Autodesk Fusion 360 part; units mm, degrees
(part 2 of 4)
sketch "Sketch4" plane through (0, 20, 0) normal (0, 1, 0) x (-1, 0, 0)
  line L0 (95, -45) -> (95, 155)
  line L1 (95, 155) -> (-95, 155)
  line L2 (-95, 155) -> (-95, -45)
  line L3 (-95, -45) -> (95, -45)
  line L4 (-63.1566, 125.0807) -> (-65.6424, 118.6138)
  line L5 (-65.6424, 118.6138) -> (-72.4858, 117.5331)
  line L6 (-72.4858, 117.5331) -> (-76.8434, 122.9193)
  line L7 (-76.8434, 122.9193) -> (-74.3576, 129.3862)
  line L8 (-74.3576, 129.3862) -> (-67.5142, 130.4669)
  line L9 (-67.5142, 130.4669) -> (-63.1566, 125.0807)
  line L10 (-63.1566, 93.0807) -> (-65.6424, 86.6138)
  line L11 (-65.6424, 86.6138) -> (-72.4858, 85.5331)
  line L12 (-72.4858, 85.5331) -> (-76.8434, 90.9193)
  line L13 (-76.8434, 90.9193) -> (-74.3576, 97.3862)
  line L14 (-74.3576, 97.3862) -> (-67.5142, 98.4669)
  line L15 (-67.5142, 98.4669) -> (-63.1566, 93.0807)
  line L16 (-63.1566, 61.0807) -> (-65.6424, 54.6138)
  line L17 (-65.6424, 54.6138) -> (-72.4858, 53.5331)
  line L18 (-72.4858, 53.5331) -> (-76.8434, 58.9193)
  line L19 (-76.8434, 58.9193) -> (-74.3576, 65.3862)
  line L20 (-74.3576, 65.3862) -> (-67.5142, 66.4669)
  line L21 (-67.5142, 66.4669) -> (-63.1566, 61.0807)
  line L22 (-63.1566, 29.0807) -> (-65.6424, 22.6138)
  line L23 (-65.6424, 22.6138) -> (-72.4858, 21.5331)
  line L24 (-72.4858, 21.5331) -> (-76.8434, 26.9193)
  line L25 (-76.8434, 26.9193) -> (-74.3576, 33.3862)
  line L26 (-74.3576, 33.3862) -> (-67.5142, 34.4669)
  line L27 (-67.5142, 34.4669) -> (-63.1566, 29.0807)
  line L28 (-63.1566, -2.9193) -> (-65.6424, -9.3862)
  line L29 (-65.6424, -9.3862) -> (-72.4858, -10.4669)
  line L30 (-72.4858, -10.4669) -> (-76.8434, -5.0807)
  line L31 (-76.8434, -5.0807) -> (-74.3576, 1.3862)
  line L32 (-74.3576, 1.3862) -> (-67.5142, 2.4669)
  line L33 (-67.5142, 2.4669) -> (-63.1566, -2.9193)
  line L34 (-49.8233, 141.0807) -> (-52.3091, 134.6138)
  line L35 (-52.3091, 134.6138) -> (-59.1525, 133.5331)
  line L36 (-59.1525, 133.5331) -> (-63.5101, 138.9193)
  line L37 (-63.5101, 138.9193) -> (-61.0243, 145.3862)
  line L38 (-61.0243, 145.3862) -> (-54.1809, 146.4669)
  line L39 (-54.1809, 146.4669) -> (-49.8233, 141.0807)
  line L40 (-49.8233, 109.0807) -> (-52.3091, 102.6138)
  line L41 (-52.3091, 102.6138) -> (-59.1525, 101.5331)
  line L42 (-59.1525, 101.5331) -> (-63.5101, 106.9193)
  line L43 (-63.5101, 106.9193) -> (-61.0243, 113.3862)
  line L44 (-61.0243, 113.3862) -> (-54.1809, 114.4669)
  line L45 (-54.1809, 114.4669) -> (-49.8233, 109.0807)
  line L46 (-49.8233, 77.0807) -> (-52.3091, 70.6138)
  line L47 (-52.3091, 70.6138) -> (-59.1525, 69.5331)
  line L48 (-59.1525, 69.5331) -> (-63.5101, 74.9193)
  line L49 (-63.5101, 74.9193) -> (-61.0243, 81.3862)
  line L50 (-61.0243, 81.3862) -> (-54.1809, 82.4669)
  line L51 (-54.1809, 82.4669) -> (-49.8233, 77.0807)
  line L52 (-49.8233, 45.0807) -> (-52.3091, 38.6138)
  line L53 (-52.3091, 38.6138) -> (-59.1525, 37.5331)
  line L54 (-59.1525, 37.5331) -> (-63.5101, 42.9193)
  line L55 (-63.5101, 42.9193) -> (-61.0243, 49.3862)
  line L56 (-61.0243, 49.3862) -> (-54.1809, 50.4669)
  line L57 (-54.1809, 50.4669) -> (-49.8233, 45.0807)
  line L58 (-49.8233, 13.0807) -> (-52.3091, 6.6138)
  line L59 (-52.3091, 6.6138) -> (-59.1525, 5.5331)
  line L60 (-59.1525, 5.5331) -> (-63.5101, 10.9193)
  line L61 (-63.5101, 10.9193) -> (-61.0243, 17.3862)
  line L62 (-61.0243, 17.3862) -> (-54.1809, 18.4669)
  line L63 (-54.1809, 18.4669) -> (-49.8233, 13.0807)
  line L64 (-49.8233, -18.9193) -> (-52.3091, -25.3862)
  line L65 (-52.3091, -25.3862) -> (-59.1525, -26.4669)
  line L66 (-59.1525, -26.4669) -> (-63.5101, -21.0807)
  line L67 (-63.5101, -21.0807) -> (-61.0243, -14.6138)
  line L68 (-61.0243, -14.6138) -> (-54.1809, -13.5331)
  line L69 (-54.1809, -13.5331) -> (-49.8233, -18.9193)
  line L70 (-36.4899, 125.0807) -> (-38.9757, 118.6138)
  line L71 (-38.9757, 118.6138) -> (-45.8191, 117.5331)
  line L72 (-45.8191, 117.5331) -> (-50.1767, 122.9193)
  line L73 (-50.1767, 122.9193) -> (-47.6909, 129.3862)
  line L74 (-47.6909, 129.3862) -> (-40.8475, 130.4669)
  line L75 (-40.8475, 130.4669) -> (-36.4899, 125.0807)
  line L76 (-36.4899, 93.0807) -> (-38.9757, 86.6138)
  line L77 (-38.9757, 86.6138) -> (-45.8191, 85.5331)
  line L78 (-45.8191, 85.5331) -> (-50.1767, 90.9193)
  line L79 (-50.1767, 90.9193) -> (-47.6909, 97.3862)
  line L80 (-47.6909, 97.3862) -> (-40.8475, 98.4669)
  line L81 (-40.8475, 98.4669) -> (-36.4899, 93.0807)
  line L82 (-36.4899, 61.0807) -> (-38.9757, 54.6138)
  line L83 (-38.9757, 54.6138) -> (-45.8191, 53.5331)
  line L84 (-45.8191, 53.5331) -> (-50.1767, 58.9193)
  line L85 (-50.1767, 58.9193) -> (-47.6909, 65.3862)
  line L86 (-47.6909, 65.3862) -> (-40.8475, 66.4669)
  line L87 (-40.8475, 66.4669) -> (-36.4899, 61.0807)
  line L88 (-36.4899, 29.0807) -> (-38.9757, 22.6138)
  line L89 (-38.9757, 22.6138) -> (-45.8191, 21.5331)
  line L90 (-45.8191, 21.5331) -> (-50.1767, 26.9193)
  line L91 (-50.1767, 26.9193) -> (-47.6909, 33.3862)
  line L92 (-47.6909, 33.3862) -> (-40.8475, 34.4669)
  line L93 (-40.8475, 34.4669) -> (-36.4899, 29.0807)
  line L94 (-36.4899, -2.9193) -> (-38.9757, -9.3862)
  line L95 (-38.9757, -9.3862) -> (-45.8191, -10.4669)
  line L96 (-45.8191, -10.4669) -> (-50.1767, -5.0807)
  line L97 (-50.1767, -5.0807) -> (-47.6909, 1.3862)
  line L98 (-47.6909, 1.3862) -> (-40.8475, 2.4669)
  line L99 (-40.8475, 2.4669) -> (-36.4899, -2.9193)
  line L100 (-23.1566, 141.0807) -> (-25.6424, 134.6138)
  line L101 (-25.6424, 134.6138) -> (-32.4858, 133.5331)
  line L102 (-32.4858, 133.5331) -> (-36.8434, 138.9193)
  line L103 (-36.8434, 138.9193) -> (-34.3576, 145.3862)
  line L104 (-34.3576, 145.3862) -> (-27.5142, 146.4669)
  line L105 (-27.5142, 146.4669) -> (-23.1566, 141.0807)
  line L106 (-23.1566, 109.0807) -> (-25.6424, 102.6138)
  line L107 (-25.6424, 102.6138) -> (-32.4858, 101.5331)
  line L108 (-32.4858, 101.5331) -> (-36.8434, 106.9193)
  line L109 (-36.8434, 106.9193) -> (-34.3576, 113.3862)
  line L110 (-34.3576, 113.3862) -> (-27.5142, 114.4669)
  line L111 (-27.5142, 114.4669) -> (-23.1566, 109.0807)
  line L112 (-23.1566, 77.0807) -> (-25.6424, 70.6138)
  line L113 (-25.6424, 70.6138) -> (-32.4858, 69.5331)
  line L114 (-32.4858, 69.5331) -> (-36.8434, 74.9193)
  line L115 (-36.8434, 74.9193) -> (-34.3576, 81.3862)
  line L116 (-34.3576, 81.3862) -> (-27.5142, 82.4669)
  line L117 (-27.5142, 82.4669) -> (-23.1566, 77.0807)
  line L118 (-23.1566, 45.0807) -> (-25.6424, 38.6138)
  line L119 (-25.6424, 38.6138) -> (-32.4858, 37.5331)
  line L120 (-32.4858, 37.5331) -> (-36.8434, 42.9193)
  line L121 (-36.8434, 42.9193) -> (-34.3576, 49.3862)
  line L122 (-34.3576, 49.3862) -> (-27.5142, 50.4669)
  line L123 (-27.5142, 50.4669) -> (-23.1566, 45.0807)
  line L124 (-23.1566, 13.0807) -> (-25.6424, 6.6138)
  line L125 (-25.6424, 6.6138) -> (-32.4858, 5.5331)
  line L126 (-32.4858, 5.5331) -> (-36.8434, 10.9193)
  line L127 (-36.8434, 10.9193) -> (-34.3576, 17.3862)
  line L128 (-34.3576, 17.3862) -> (-27.5142, 18.4669)
  line L129 (-27.5142, 18.4669) -> (-23.1566, 13.0807)
  line L130 (-23.1566, -18.9193) -> (-25.6424, -25.3862)
  line L131 (-25.6424, -25.3862) -> (-32.4858, -26.4669)
  line L132 (-32.4858, -26.4669) -> (-36.8434, -21.0807)
  line L133 (-36.8434, -21.0807) -> (-34.3576, -14.6138)
  line L134 (-34.3576, -14.6138) -> (-27.5142, -13.5331)
  line L135 (-27.5142, -13.5331) -> (-23.1566, -18.9193)
  line L136 (-9.8233, 125.0807) -> (-12.3091, 118.6138)
  line L137 (-12.3091, 118.6138) -> (-19.1525, 117.5331)
  line L138 (-19.1525, 117.5331) -> (-23.5101, 122.9193)
  line L139 (-23.5101, 122.9193) -> (-21.0243, 129.3862)
  line L140 (-21.0243, 129.3862) -> (-14.1809, 130.4669)
  line L141 (-14.1809, 130.4669) -> (-9.8233, 125.0807)
  line L142 (-9.8233, 93.0807) -> (-12.3091, 86.6138)
  line L143 (-12.3091, 86.6138) -> (-19.1525, 85.5331)
  line L144 (-19.1525, 85.5331) -> (-23.5101, 90.9193)
  line L145 (-23.5101, 90.9193) -> (-21.0243, 97.3862)
  line L146 (-21.0243, 97.3862) -> (-14.1809, 98.4669)
  line L147 (-14.1809, 98.4669) -> (-9.8233, 93.0807)
  line L148 (-9.8233, 61.0807) -> (-12.3091, 54.6138)
  line L149 (-12.3091, 54.6138) -> (-19.1525, 53.5331)
  line L150 (-19.1525, 53.5331) -> (-23.5101, 58.9193)
  line L151 (-23.5101, 58.9193) -> (-21.0243, 65.3862)
  line L152 (-21.0243, 65.3862) -> (-14.1809, 66.4669)
  line L153 (-14.1809, 66.4669) -> (-9.8233, 61.0807)
  line L154 (-9.8233, 29.0807) -> (-12.3091, 22.6138)
  line L155 (-12.3091, 22.6138) -> (-19.1525, 21.5331)
  line L156 (-19.1525, 21.5331) -> (-23.5101, 26.9193)
  line L157 (-23.5101, 26.9193) -> (-21.0243, 33.3862)
  line L158 (-21.0243, 33.3862) -> (-14.1809, 34.4669)
  line L159 (-14.1809, 34.4669) -> (-9.8233, 29.0807)
  line L160 (-9.8233, -2.9193) -> (-12.3091, -9.3862)
  line L161 (-12.3091, -9.3862) -> (-19.1525, -10.4669)
  line L162 (-19.1525, -10.4669) -> (-23.5101, -5.0807)
  line L163 (-23.5101, -5.0807) -> (-21.0243, 1.3862)
  line L164 (-21.0243, 1.3862) -> (-14.1809, 2.4669)
  line L165 (-14.1809, 2.4669) -> (-9.8233, -2.9193)
  line L166 (-0.8475, 146.4669) -> (3.5101, 141.0807)
  line L167 (3.5101, 141.0807) -> (1.0243, 134.6138)
  line L168 (1.0243, 134.6138) -> (-5.8191, 133.5331)
  line L169 (-5.8191, 133.5331) -> (-10.1767, 138.9193)
  line L170 (-10.1767, 138.9193) -> (-7.6909, 145.3862)
  line L171 (-7.6909, 145.3862) -> (-0.8475, 146.4669)
  line L172 (-0.8475, 114.4669) -> (3.5101, 109.0807)
  line L173 (3.5101, 109.0807) -> (1.0243, 102.6138)
  line L174 (1.0243, 102.6138) -> (-5.8191, 101.5331)
  line L175 (-5.8191, 101.5331) -> (-10.1767, 106.9193)
  line L176 (-10.1767, 106.9193) -> (-7.6909, 113.3862)
  line L177 (-7.6909, 113.3862) -> (-0.8475, 114.4669)
  line L178 (-0.8475, 82.4669) -> (3.5101, 77.0807)
  line L179 (3.5101, 77.0807) -> (1.0243, 70.6138)
  line L180 (1.0243, 70.6138) -> (-5.8191, 69.5331)
  line L181 (-5.8191, 69.5331) -> (-10.1767, 74.9193)
  line L182 (-10.1767, 74.9193) -> (-7.6909, 81.3862)
  line L183 (-7.6909, 81.3862) -> (-0.8475, 82.4669)
  line L184 (-0.8475, 50.4669) -> (3.5101, 45.0807)
  line L185 (3.5101, 45.0807) -> (1.0243, 38.6138)
  line L186 (1.0243, 38.6138) -> (-5.8191, 37.5331)
  line L187 (-5.8191, 37.5331) -> (-10.1767, 42.9193)
  line L188 (-10.1767, 42.9193) -> (-7.6909, 49.3862)
  line L189 (-7.6909, 49.3862) -> (-0.8475, 50.4669)
  line L190 (-0.8475, 18.4669) -> (3.5101, 13.0807)
  line L191 (3.5101, 13.0807) -> (1.0243, 6.6138)
  line L192 (1.0243, 6.6138) -> (-5.8191, 5.5331)
  line L193 (-5.8191, 5.5331) -> (-10.1767, 10.9193)
  line L194 (-10.1767, 10.9193) -> (-7.6909, 17.3862)
  line L195 (-7.6909, 17.3862) -> (-0.8475, 18.4669)
  line L196 (-0.8475, -13.5331) -> (3.5101, -18.9193)
  line L197 (3.5101, -18.9193) -> (1.0243, -25.3862)
  line L198 (1.0243, -25.3862) -> (-5.8191, -26.4669)
  line L199 (-5.8191, -26.4669) -> (-10.1767, -21.0807)
  line L200 (-10.1767, -21.0807) -> (-7.6909, -14.6138)
  line L201 (-7.6909, -14.6138) -> (-0.8475, -13.5331)
  line L202 (12.4858, 130.4669) -> (16.8434, 125.0807)
  line L203 (16.8434, 125.0807) -> (14.3576, 118.6138)
  line L204 (14.3576, 118.6138) -> (7.5142, 117.5331)
  line L205 (7.5142, 117.5331) -> (3.1566, 122.9193)
  line L206 (3.1566, 122.9193) -> (5.6424, 129.3862)
  line L207 (5.6424, 129.3862) -> (12.4858, 130.4669)
  line L208 (12.4858, 98.4669) -> (16.8434, 93.0807)
  line L209 (16.8434, 93.0807) -> (14.3576, 86.6138)
  line L210 (14.3576, 86.6138) -> (7.5142, 85.5331)
  line L211 (7.5142, 85.5331) -> (3.1566, 90.9193)
  line L212 (3.1566, 90.9193) -> (5.6424, 97.3862)
  line L213 (5.6424, 97.3862) -> (12.4858, 98.4669)
  line L214 (12.4858, 66.4669) -> (16.8434, 61.0807)
  line L215 (16.8434, 61.0807) -> (14.3576, 54.6138)
  line L216 (14.3576, 54.6138) -> (7.5142, 53.5331)
  line L217 (7.5142, 53.5331) -> (3.1566, 58.9193)
  line L218 (3.1566, 58.9193) -> (5.6424, 65.3862)
  line L219 (5.6424, 65.3862) -> (12.4858, 66.4669)
  line L220 (12.4858, 34.4669) -> (16.8434, 29.0807)
  line L221 (16.8434, 29.0807) -> (14.3576, 22.6138)
  line L222 (14.3576, 22.6138) -> (7.5142, 21.5331)
  line L223 (7.5142, 21.5331) -> (3.1566, 26.9193)
  line L224 (3.1566, 26.9193) -> (5.6424, 33.3862)
  line L225 (5.6424, 33.3862) -> (12.4858, 34.4669)
  line L226 (12.4858, 2.4669) -> (16.8434, -2.9193)
  line L227 (16.8434, -2.9193) -> (14.3576, -9.3862)
  line L228 (14.3576, -9.3862) -> (7.5142, -10.4669)
  line L229 (7.5142, -10.4669) -> (3.1566, -5.0807)
  line L230 (3.1566, -5.0807) -> (5.6424, 1.3862)
  line L231 (5.6424, 1.3862) -> (12.4858, 2.4669)
  line L232 (25.8191, 146.4669) -> (30.1767, 141.0807)
  line L233 (30.1767, 141.0807) -> (27.6909, 134.6138)
  line L234 (27.6909, 134.6138) -> (20.8475, 133.5331)
  line L235 (20.8475, 133.5331) -> (16.4899, 138.9193)
  line L236 (16.4899, 138.9193) -> (18.9757, 145.3862)
  line L237 (18.9757, 145.3862) -> (25.8191, 146.4669)
  line L238 (25.8191, 114.4669) -> (30.1767, 109.0807)
  line L239 (30.1767, 109.0807) -> (27.6909, 102.6138)
  line L240 (27.6909, 102.6138) -> (20.8475, 101.5331)
  line L241 (20.8475, 101.5331) -> (16.4899, 106.9193)
  line L242 (16.4899, 106.9193) -> (18.9757, 113.3862)
  line L243 (18.9757, 113.3862) -> (25.8191, 114.4669)
  line L244 (25.8191, 82.4669) -> (30.1767, 77.0807)
  line L245 (30.1767, 77.0807) -> (27.6909, 70.6138)
  line L246 (27.6909, 70.6138) -> (20.8475, 69.5331)
  line L247 (20.8475, 69.5331) -> (16.4899, 74.9193)
  line L248 (16.4899, 74.9193) -> (18.9757, 81.3862)
  line L249 (18.9757, 81.3862) -> (25.8191, 82.4669)
  line L250 (25.8191, 50.4669) -> (30.1767, 45.0807)
  line L251 (30.1767, 45.0807) -> (27.6909, 38.6138)
  line L252 (27.6909, 38.6138) -> (20.8475, 37.5331)
  line L253 (20.8475, 37.5331) -> (16.4899, 42.9193)
  line L254 (16.4899, 42.9193) -> (18.9757, 49.3862)
  line L255 (18.9757, 49.3862) -> (25.8191, 50.4669)
  line L256 (25.8191, 18.4669) -> (30.1767, 13.0807)
  line L257 (30.1767, 13.0807) -> (27.6909, 6.6138)
  line L258 (27.6909, 6.6138) -> (20.8475, 5.5331)
  line L259 (20.8475, 5.5331) -> (16.4899, 10.9193)
  line L260 (16.4899, 10.9193) -> (18.9757, 17.3862)
  line L261 (18.9757, 17.3862) -> (25.8191, 18.4669)
  line L262 (25.8191, -13.5331) -> (30.1767, -18.9193)
  line L263 (30.1767, -18.9193) -> (27.6909, -25.3862)
  line L264 (27.6909, -25.3862) -> (20.8475, -26.4669)
  line L265 (20.8475, -26.4669) -> (16.4899, -21.0807)
  line L266 (16.4899, -21.0807) -> (18.9757, -14.6138)
  line L267 (18.9757, -14.6138) -> (25.8191, -13.5331)
  line L268 (39.1525, 130.4669) -> (43.5101, 125.0807)
  line L269 (43.5101, 125.0807) -> (41.0243, 118.6138)
  line L270 (41.0243, 118.6138) -> (34.1809, 117.5331)
  line L271 (34.1809, 117.5331) -> (29.8233, 122.9193)
  line L272 (29.8233, 122.9193) -> (32.3091, 129.3862)
  line L273 (32.3091, 129.3862) -> (39.1525, 130.4669)
  line L274 (39.1525, 98.4669) -> (43.5101, 93.0807)
  line L275 (43.5101, 93.0807) -> (41.0243, 86.6138)
  line L276 (41.0243, 86.6138) -> (34.1809, 85.5331)
  line L277 (34.1809, 85.5331) -> (29.8233, 90.9193)
  line L278 (29.8233, 90.9193) -> (32.3091, 97.3862)
  line L279 (32.3091, 97.3862) -> (39.1525, 98.4669)
  line L280 (39.1525, 66.4669) -> (43.5101, 61.0807)
  line L281 (43.5101, 61.0807) -> (41.0243, 54.6138)
  line L282 (41.0243, 54.6138) -> (34.1809, 53.5331)
  line L283 (34.1809, 53.5331) -> (29.8233, 58.9193)
  line L284 (29.8233, 58.9193) -> (32.3091, 65.3862)
  line L285 (32.3091, 65.3862) -> (39.1525, 66.4669)
  line L286 (39.1525, 34.4669) -> (43.5101, 29.0807)
  line L287 (43.5101, 29.0807) -> (41.0243, 22.6138)
  line L288 (41.0243, 22.6138) -> (34.1809, 21.5331)
  line L289 (34.1809, 21.5331) -> (29.8233, 26.9193)
  line L290 (29.8233, 26.9193) -> (32.3091, 33.3862)
  line L291 (32.3091, 33.3862) -> (39.1525, 34.4669)
  line L292 (39.1525, 2.4669) -> (43.5101, -2.9193)
  line L293 (43.5101, -2.9193) -> (41.0243, -9.3862)
  line L294 (41.0243, -9.3862) -> (34.1809, -10.4669)
  line L295 (34.1809, -10.4669) -> (29.8233, -5.0807)
  line L296 (29.8233, -5.0807) -> (32.3091, 1.3862)
  line L297 (32.3091, 1.3862) -> (39.1525, 2.4669)
  line L298 (52.4858, 146.4669) -> (56.8434, 141.0807)
  line L299 (56.8434, 141.0807) -> (54.3576, 134.6138)
  line L300 (54.3576, 134.6138) -> (47.5142, 133.5331)
  line L301 (47.5142, 133.5331) -> (43.1566, 138.9193)
  line L302 (43.1566, 138.9193) -> (45.6424, 145.3862)
  line L303 (45.6424, 145.3862) -> (52.4858, 146.4669)
  line L304 (52.4858, 114.4669) -> (56.8434, 109.0807)
  line L305 (56.8434, 109.0807) -> (54.3576, 102.6138)
  line L306 (54.3576, 102.6138) -> (47.5142, 101.5331)
  line L307 (47.5142, 101.5331) -> (43.1566, 106.9193)
  line L308 (43.1566, 106.9193) -> (45.6424, 113.3862)
  line L309 (45.6424, 113.3862) -> (52.4858, 114.4669)
  line L310 (52.4858, 82.4669) -> (56.8434, 77.0807)
  line L311 (56.8434, 77.0807) -> (54.3576, 70.6138)
  line L312 (54.3576, 70.6138) -> (47.5142, 69.5331)
  line L313 (47.5142, 69.5331) -> (43.1566, 74.9193)
  line L314 (43.1566, 74.9193) -> (45.6424, 81.3862)
  line L315 (45.6424, 81.3862) -> (52.4858, 82.4669)
  line L316 (52.4858, 50.4669) -> (56.8434, 45.0807)
  line L317 (56.8434, 45.0807) -> (54.3576, 38.6138)
  line L318 (54.3576, 38.6138) -> (47.5142, 37.5331)
  line L319 (47.5142, 37.5331) -> (43.1566, 42.9193)
  line L320 (43.1566, 42.9193) -> (45.6424, 49.3862)
  line L321 (45.6424, 49.3862) -> (52.4858, 50.4669)
  line L322 (52.4858, 18.4669) -> (56.8434, 13.0807)
  line L323 (56.8434, 13.0807) -> (54.3576, 6.6138)
  line L324 (54.3576, 6.6138) -> (47.5142, 5.5331)
  line L325 (47.5142, 5.5331) -> (43.1566, 10.9193)
  line L326 (43.1566, 10.9193) -> (45.6424, 17.3862)
  line L327 (45.6424, 17.3862) -> (52.4858, 18.4669)
  line L328 (47.5142, -26.4669) -> (43.1566, -21.0807)
  line L329 (43.1566, -21.0807) -> (45.6424, -14.6138)
  line L330 (45.6424, -14.6138) -> (52.4858, -13.5331)
  line L331 (52.4858, -13.5331) -> (56.8434, -18.9193)
  line L332 (56.8434, -18.9193) -> (54.3576, -25.3862)
  line L333 (54.3576, -25.3862) -> (47.5142, -26.4669)
  line L334 (52.4858, 2.4669) -> (56.8434, -2.9193)
  line L335 (56.8434, -2.9193) -> (54.3576, -9.3862)
  line L336 (54.3576, -9.3862) -> (47.5142, -10.4669)
  line L337 (47.5142, -10.4669) -> (43.1566, -5.0807)
  line L338 (43.1566, -5.0807) -> (45.6424, 1.3862)
  line L339 (45.6424, 1.3862) -> (52.4858, 2.4669)
  line L340 (52.4858, 34.4669) -> (56.8434, 29.0807)
  line L341 (56.8434, 29.0807) -> (54.3576, 22.6138)
  line L342 (54.3576, 22.6138) -> (47.5142, 21.5331)
  line L343 (47.5142, 21.5331) -> (43.1566, 26.9193)
  line L344 (43.1566, 26.9193) -> (45.6424, 33.3862)
  line L345 (45.6424, 33.3862) -> (52.4858, 34.4669)
  line L346 (52.4858, 66.4669) -> (56.8434, 61.0807)
  line L347 (56.8434, 61.0807) -> (54.3576, 54.6138)
  line L348 (54.3576, 54.6138) -> (47.5142, 53.5331)
  line L349 (47.5142, 53.5331) -> (43.1566, 58.9193)
  line L350 (43.1566, 58.9193) -> (45.6424, 65.3862)
  line L351 (45.6424, 65.3862) -> (52.4858, 66.4669)
  line L352 (52.4858, 98.4669) -> (56.8434, 93.0807)
  line L353 (56.8434, 93.0807) -> (54.3576, 86.6138)
  line L354 (54.3576, 86.6138) -> (47.5142, 85.5331)
  line L355 (47.5142, 85.5331) -> (43.1566, 90.9193)
  line L356 (43.1566, 90.9193) -> (45.6424, 97.3862)
  line L357 (45.6424, 97.3862) -> (52.4858, 98.4669)
  line L358 (52.4858, 130.4669) -> (56.8434, 125.0807)
  line L359 (56.8434, 125.0807) -> (54.3576, 118.6138)
  line L360 (54.3576, 118.6138) -> (47.5142, 117.5331)
  line L361 (47.5142, 117.5331) -> (43.1566, 122.9193)
  line L362 (43.1566, 122.9193) -> (45.6424, 129.3862)
  line L363 (45.6424, 129.3862) -> (52.4858, 130.4669)
  line L364 (39.1525, -13.5331) -> (43.5101, -18.9193)
  line L365 (43.5101, -18.9193) -> (41.0243, -25.3862)
  line L366 (41.0243, -25.3862) -> (34.1809, -26.4669)
  line L367 (34.1809, -26.4669) -> (29.8233, -21.0807)
  line L368 (29.8233, -21.0807) -> (32.3091, -14.6138)
  line L369 (32.3091, -14.6138) -> (39.1525, -13.5331)
  line L370 (39.1525, 18.4669) -> (43.5101, 13.0807)
  line L371 (43.5101, 13.0807) -> (41.0243, 6.6138)
  line L372 (41.0243, 6.6138) -> (34.1809, 5.5331)
  line L373 (34.1809, 5.5331) -> (29.8233, 10.9193)
  line L374 (29.8233, 10.9193) -> (32.3091, 17.3862)
  line L375 (32.3091, 17.3862) -> (39.1525, 18.4669)
  line L376 (39.1525, 50.4669) -> (43.5101, 45.0807)
  line L377 (43.5101, 45.0807) -> (41.0243, 38.6138)
  line L378 (41.0243, 38.6138) -> (34.1809, 37.5331)
  line L379 (34.1809, 37.5331) -> (29.8233, 42.9193)
  line L380 (29.8233, 42.9193) -> (32.3091, 49.3862)
  line L381 (32.3091, 49.3862) -> (39.1525, 50.4669)
  line L382 (39.1525, 82.4669) -> (43.5101, 77.0807)
  line L383 (43.5101, 77.0807) -> (41.0243, 70.6138)
  line L384 (41.0243, 70.6138) -> (34.1809, 69.5331)
  line L385 (34.1809, 69.5331) -> (29.8233, 74.9193)
  line L386 (29.8233, 74.9193) -> (32.3091, 81.3862)
  line L387 (32.3091, 81.3862) -> (39.1525, 82.4669)
  line L388 (39.1525, 114.4669) -> (43.5101, 109.0807)
  line L389 (43.5101, 109.0807) -> (41.0243, 102.6138)
  line L390 (41.0243, 102.6138) -> (34.1809, 101.5331)
  line L391 (34.1809, 101.5331) -> (29.8233, 106.9193)
  line L392 (29.8233, 106.9193) -> (32.3091, 113.3862)
  line L393 (32.3091, 113.3862) -> (39.1525, 114.4669)
  line L394 (39.1525, 146.4669) -> (43.5101, 141.0807)
  line L395 (43.5101, 141.0807) -> (41.0243, 134.6138)
  line L396 (41.0243, 134.6138) -> (34.1809, 133.5331)
  line L397 (34.1809, 133.5331) -> (29.8233, 138.9193)
  line L398 (29.8233, 138.9193) -> (32.3091, 145.3862)
  line L399 (32.3091, 145.3862) -> (39.1525, 146.4669)
  line L400 (25.8191, 2.4669) -> (30.1767, -2.9193)
  line L401 (30.1767, -2.9193) -> (27.6909, -9.3862)
  line L402 (27.6909, -9.3862) -> (20.8475, -10.4669)
  line L403 (20.8475, -10.4669) -> (16.4899, -5.0807)
  line L404 (16.4899, -5.0807) -> (18.9757, 1.3862)
  line L405 (18.9757, 1.3862) -> (25.8191, 2.4669)
  line L406 (25.8191, 34.4669) -> (30.1767, 29.0807)
  line L407 (30.1767, 29.0807) -> (27.6909, 22.6138)
  line L408 (27.6909, 22.6138) -> (20.8475, 21.5331)
  line L409 (20.8475, 21.5331) -> (16.4899, 26.9193)
  line L410 (16.4899, 26.9193) -> (18.9757, 33.3862)
  line L411 (18.9757, 33.3862) -> (25.8191, 34.4669)
  line L412 (25.8191, 66.4669) -> (30.1767, 61.0807)
  line L413 (30.1767, 61.0807) -> (27.6909, 54.6138)
  line L414 (27.6909, 54.6138) -> (20.8475, 53.5331)
  line L415 (20.8475, 53.5331) -> (16.4899, 58.9193)
  line L416 (16.4899, 58.9193) -> (18.9757, 65.3862)
  line L417 (18.9757, 65.3862) -> (25.8191, 66.4669)
  line L418 (25.8191, 98.4669) -> (30.1767, 93.0807)
  line L419 (30.1767, 93.0807) -> (27.6909, 86.6138)
  line L420 (27.6909, 86.6138) -> (20.8475, 85.5331)
  line L421 (20.8475, 85.5331) -> (16.4899, 90.9193)
  line L422 (16.4899, 90.9193) -> (18.9757, 97.3862)
  line L423 (18.9757, 97.3862) -> (25.8191, 98.4669)
  line L424 (25.8191, 130.4669) -> (30.1767, 125.0807)
  line L425 (30.1767, 125.0807) -> (27.6909, 118.6138)
  line L426 (27.6909, 118.6138) -> (20.8475, 117.5331)
  line L427 (20.8475, 117.5331) -> (16.4899, 122.9193)
  line L428 (16.4899, 122.9193) -> (18.9757, 129.3862)
  line L429 (18.9757, 129.3862) -> (25.8191, 130.4669)
  line L430 (12.4858, -13.5331) -> (16.8434, -18.9193)
  line L431 (16.8434, -18.9193) -> (14.3576, -25.3862)
  line L432 (14.3576, -25.3862) -> (7.5142, -26.4669)
  line L433 (7.5142, -26.4669) -> (3.1566, -21.0807)
  line L434 (3.1566, -21.0807) -> (5.6424, -14.6138)
  line L435 (5.6424, -14.6138) -> (12.4858, -13.5331)
  line L436 (12.4858, 18.4669) -> (16.8434, 13.0807)
  line L437 (16.8434, 13.0807) -> (14.3576, 6.6138)
  line L438 (14.3576, 6.6138) -> (7.5142, 5.5331)
  line L439 (7.5142, 5.5331) -> (3.1566, 10.9193)
  line L440 (3.1566, 10.9193) -> (5.6424, 17.3862)
  line L441 (5.6424, 17.3862) -> (12.4858, 18.4669)
  line L442 (12.4858, 50.4669) -> (16.8434, 45.0807)
  line L443 (16.8434, 45.0807) -> (14.3576, 38.6138)
  line L444 (14.3576, 38.6138) -> (7.5142, 37.5331)
  line L445 (7.5142, 37.5331) -> (3.1566, 42.9193)
  line L446 (3.1566, 42.9193) -> (5.6424, 49.3862)
  line L447 (5.6424, 49.3862) -> (12.4858, 50.4669)
  line L448 (12.4858, 82.4669) -> (16.8434, 77.0807)
  line L449 (16.8434, 77.0807) -> (14.3576, 70.6138)
  line L450 (14.3576, 70.6138) -> (7.5142, 69.5331)
  line L451 (7.5142, 69.5331) -> (3.1566, 74.9193)
  line L452 (3.1566, 74.9193) -> (5.6424, 81.3862)
  line L453 (5.6424, 81.3862) -> (12.4858, 82.4669)
  line L454 (12.4858, 114.4669) -> (16.8434, 109.0807)
  line L455 (16.8434, 109.0807) -> (14.3576, 102.6138)
  line L456 (14.3576, 102.6138) -> (7.5142, 101.5331)
  line L457 (7.5142, 101.5331) -> (3.1566, 106.9193)
  line L458 (3.1566, 106.9193) -> (5.6424, 113.3862)
  line L459 (5.6424, 113.3862) -> (12.4858, 114.4669)
  line L460 (12.4858, 146.4669) -> (16.8434, 141.0807)
  line L461 (16.8434, 141.0807) -> (14.3576, 134.6138)
  line L462 (14.3576, 134.6138) -> (7.5142, 133.5331)
  line L463 (7.5142, 133.5331) -> (3.1566, 138.9193)
  line L464 (3.1566, 138.9193) -> (5.6424, 145.3862)
  line L465 (5.6424, 145.3862) -> (12.4858, 146.4669)
  line L466 (-0.8475, 2.4669) -> (3.5101, -2.9193)
  line L467 (3.5101, -2.9193) -> (1.0243, -9.3862)
  line L468 (1.0243, -9.3862) -> (-5.8191, -10.4669)
  line L469 (-5.8191, -10.4669) -> (-10.1767, -5.0807)
  line L470 (-10.1767, -5.0807) -> (-7.6909, 1.3862)
  line L471 (-7.6909, 1.3862) -> (-0.8475, 2.4669)
  line L472 (-0.8475, 34.4669) -> (3.5101, 29.0807)
  line L473 (3.5101, 29.0807) -> (1.0243, 22.6138)
  line L474 (1.0243, 22.6138) -> (-5.8191, 21.5331)
  line L475 (-5.8191, 21.5331) -> (-10.1767, 26.9193)
  line L476 (-10.1767, 26.9193) -> (-7.6909, 33.3862)
  line L477 (-7.6909, 33.3862) -> (-0.8475, 34.4669)
  line L478 (-0.8475, 66.4669) -> (3.5101, 61.0807)
  line L479 (3.5101, 61.0807) -> (1.0243, 54.6138)
  line L480 (1.0243, 54.6138) -> (-5.8191, 53.5331)
  line L481 (-5.8191, 53.5331) -> (-10.1767, 58.9193)
  line L482 (-10.1767, 58.9193) -> (-7.6909, 65.3862)
  line L483 (-7.6909, 65.3862) -> (-0.8475, 66.4669)
  line L484 (-0.8475, 98.4669) -> (3.5101, 93.0807)
  line L485 (3.5101, 93.0807) -> (1.0243, 86.6138)
  line L486 (1.0243, 86.6138) -> (-5.8191, 85.5331)
  line L487 (-5.8191, 85.5331) -> (-10.1767, 90.9193)
  line L488 (-10.1767, 90.9193) -> (-7.6909, 97.3862)
  line L489 (-7.6909, 97.3862) -> (-0.8475, 98.4669)
  line L490 (-0.8475, 130.4669) -> (3.5101, 125.0807)
  line L491 (3.5101, 125.0807) -> (1.0243, 118.6138)
  line L492 (1.0243, 118.6138) -> (-5.8191, 117.5331)
  line L493 (-5.8191, 117.5331) -> (-10.1767, 122.9193)
  line L494 (-10.1767, 122.9193) -> (-7.6909, 129.3862)
  line L495 (-7.6909, 129.3862) -> (-0.8475, 130.4669)
  line L496 (-14.1809, -13.5331) -> (-9.8233, -18.9193)
  line L497 (-9.8233, -18.9193) -> (-12.3091, -25.3862)
  line L498 (-12.3091, -25.3862) -> (-19.1525, -26.4669)
  line L499 (-19.1525, -26.4669) -> (-23.5101, -21.0807)
  line L500 (-23.5101, -21.0807) -> (-21.0243, -14.6138)
  line L501 (-21.0243, -14.6138) -> (-14.1809, -13.5331)
  line L502 (-9.8233, 13.0807) -> (-12.3091, 6.6138)
  line L503 (-12.3091, 6.6138) -> (-19.1525, 5.5331)
  line L504 (-19.1525, 5.5331) -> (-23.5101, 10.9193)
  line L505 (-23.5101, 10.9193) -> (-21.0243, 17.3862)
  line L506 (-21.0243, 17.3862) -> (-14.1809, 18.4669)
  line L507 (-14.1809, 18.4669) -> (-9.8233, 13.0807)
  line L508 (-9.8233, 45.0807) -> (-12.3091, 38.6138)
  line L509 (-12.3091, 38.6138) -> (-19.1525, 37.5331)
  line L510 (-19.1525, 37.5331) -> (-23.5101, 42.9193)
  line L511 (-23.5101, 42.9193) -> (-21.0243, 49.3862)
  line L512 (-21.0243, 49.3862) -> (-14.1809, 50.4669)
  line L513 (-14.1809, 50.4669) -> (-9.8233, 45.0807)
  line L514 (-9.8233, 77.0807) -> (-12.3091, 70.6138)
  line L515 (-12.3091, 70.6138) -> (-19.1525, 69.5331)
  line L516 (-19.1525, 69.5331) -> (-23.5101, 74.9193)
  line L517 (-23.5101, 74.9193) -> (-21.0243, 81.3862)
  line L518 (-21.0243, 81.3862) -> (-14.1809, 82.4669)
  line L519 (-14.1809, 82.4669) -> (-9.8233, 77.0807)
  line L520 (-9.8233, 109.0807) -> (-12.3091, 102.6138)
  line L521 (-12.3091, 102.6138) -> (-19.1525, 101.5331)
  line L522 (-19.1525, 101.5331) -> (-23.5101, 106.9193)
  line L523 (-23.5101, 106.9193) -> (-21.0243, 113.3862)
  line L524 (-21.0243, 113.3862) -> (-14.1809, 114.4669)
  line L525 (-14.1809, 114.4669) -> (-9.8233, 109.0807)
  line L526 (-9.8233, 141.0807) -> (-12.3091, 134.6138)
  line L527 (-12.3091, 134.6138) -> (-19.1525, 133.5331)
  line L528 (-19.1525, 133.5331) -> (-23.5101, 138.9193)
  line L529 (-23.5101, 138.9193) -> (-21.0243, 145.3862)
  line L530 (-21.0243, 145.3862) -> (-14.1809, 146.4669)
  line L531 (-14.1809, 146.4669) -> (-9.8233, 141.0807)
  line L532 (-23.1566, -2.9193) -> (-25.6424, -9.3862)
  line L533 (-25.6424, -9.3862) -> (-32.4858, -10.4669)
  line L534 (-32.4858, -10.4669) -> (-36.8434, -5.0807)
  line L535 (-36.8434, -5.0807) -> (-34.3576, 1.3862)
  line L536 (-34.3576, 1.3862) -> (-27.5142, 2.4669)
  line L537 (-27.5142, 2.4669) -> (-23.1566, -2.9193)
  line L538 (-23.1566, 29.0807) -> (-25.6424, 22.6138)
  line L539 (-25.6424, 22.6138) -> (-32.4858, 21.5331)
  line L540 (-32.4858, 21.5331) -> (-36.8434, 26.9193)
  line L541 (-36.8434, 26.9193) -> (-34.3576, 33.3862)
  line L542 (-34.3576, 33.3862) -> (-27.5142, 34.4669)
  line L543 (-27.5142, 34.4669) -> (-23.1566, 29.0807)
  line L544 (-23.1566, 61.0807) -> (-25.6424, 54.6138)
  line L545 (-25.6424, 54.6138) -> (-32.4858, 53.5331)
  line L546 (-32.4858, 53.5331) -> (-36.8434, 58.9193)
  line L547 (-36.8434, 58.9193) -> (-34.3576, 65.3862)
  line L548 (-34.3576, 65.3862) -> (-27.5142, 66.4669)
  line L549 (-27.5142, 66.4669) -> (-23.1566, 61.0807)
  line L550 (-23.1566, 93.0807) -> (-25.6424, 86.6138)
  line L551 (-25.6424, 86.6138) -> (-32.4858, 85.5331)
  line L552 (-32.4858, 85.5331) -> (-36.8434, 90.9193)
  line L553 (-36.8434, 90.9193) -> (-34.3576, 97.3862)
  line L554 (-34.3576, 97.3862) -> (-27.5142, 98.4669)
  line L555 (-27.5142, 98.4669) -> (-23.1566, 93.0807)
  line L556 (-23.1566, 125.0807) -> (-25.6424, 118.6138)
  line L557 (-25.6424, 118.6138) -> (-32.4858, 117.5331)
  line L558 (-32.4858, 117.5331) -> (-36.8434, 122.9193)
  line L559 (-36.8434, 122.9193) -> (-34.3576, 129.3862)
  line L560 (-34.3576, 129.3862) -> (-27.5142, 130.4669)
  line L561 (-27.5142, 130.4669) -> (-23.1566, 125.0807)
  line L562 (-36.4899, -18.9193) -> (-38.9757, -25.3862)
  line L563 (-38.9757, -25.3862) -> (-45.8191, -26.4669)
  line L564 (-45.8191, -26.4669) -> (-50.1767, -21.0807)
  line L565 (-50.1767, -21.0807) -> (-47.6909, -14.6138)
  line L566 (-47.6909, -14.6138) -> (-40.8475, -13.5331)
  line L567 (-40.8475, -13.5331) -> (-36.4899, -18.9193)
  line L568 (-36.4899, 13.0807) -> (-38.9757, 6.6138)
  line L569 (-38.9757, 6.6138) -> (-45.8191, 5.5331)
  line L570 (-45.8191, 5.5331) -> (-50.1767, 10.9193)
  line L571 (-50.1767, 10.9193) -> (-47.6909, 17.3862)
  line L572 (-47.6909, 17.3862) -> (-40.8475, 18.4669)
  line L573 (-40.8475, 18.4669) -> (-36.4899, 13.0807)
  line L574 (-36.4899, 45.0807) -> (-38.9757, 38.6138)
  line L575 (-38.9757, 38.6138) -> (-45.8191, 37.5331)
  line L576 (-45.8191, 37.5331) -> (-50.1767, 42.9193)
  line L577 (-50.1767, 42.9193) -> (-47.6909, 49.3862)
  line L578 (-47.6909, 49.3862) -> (-40.8475, 50.4669)
  line L579 (-40.8475, 50.4669) -> (-36.4899, 45.0807)
  line L580 (-36.4899, 77.0807) -> (-38.9757, 70.6138)
  line L581 (-38.9757, 70.6138) -> (-45.8191, 69.5331)
  line L582 (-45.8191, 69.5331) -> (-50.1767, 74.9193)
  line L583 (-50.1767, 74.9193) -> (-47.6909, 81.3862)
  line L584 (-47.6909, 81.3862) -> (-40.8475, 82.4669)
  line L585 (-40.8475, 82.4669) -> (-36.4899, 77.0807)
  line L586 (-36.4899, 109.0807) -> (-38.9757, 102.6138)
  line L587 (-38.9757, 102.6138) -> (-45.8191, 101.5331)
  line L588 (-45.8191, 101.5331) -> (-50.1767, 106.9193)
  line L589 (-50.1767, 106.9193) -> (-47.6909, 113.3862)
  line L590 (-47.6909, 113.3862) -> (-40.8475, 114.4669)
  line L591 (-40.8475, 114.4669) -> (-36.4899, 109.0807)
  line L592 (-36.4899, 141.0807) -> (-38.9757, 134.6138)
  line L593 (-38.9757, 134.6138) -> (-45.8191, 133.5331)
  line L594 (-45.8191, 133.5331) -> (-50.1767, 138.9193)
  line L595 (-50.1767, 138.9193) -> (-47.6909, 145.3862)
  line L596 (-47.6909, 145.3862) -> (-40.8475, 146.4669)
  line L597 (-40.8475, 146.4669) -> (-36.4899, 141.0807)
  line L598 (-49.8233, -2.9193) -> (-52.3091, -9.3862)
  line L599 (-52.3091, -9.3862) -> (-59.1525, -10.4669)
  line L600 (-59.1525, -10.4669) -> (-63.5101, -5.0807)
  line L601 (-63.5101, -5.0807) -> (-61.0243, 1.3862)
  line L602 (-61.0243, 1.3862) -> (-54.1809, 2.4669)
  line L603 (-54.1809, 2.4669) -> (-49.8233, -2.9193)
  line L604 (-49.8233, 29.0807) -> (-52.3091, 22.6138)
  line L605 (-52.3091, 22.6138) -> (-59.1525, 21.5331)
  line L606 (-59.1525, 21.5331) -> (-63.5101, 26.9193)
  line L607 (-63.5101, 26.9193) -> (-61.0243, 33.3862)
  line L608 (-61.0243, 33.3862) -> (-54.1809, 34.4669)
  line L609 (-54.1809, 34.4669) -> (-49.8233, 29.0807)
  line L610 (-49.8233, 61.0807) -> (-52.3091, 54.6138)
  line L611 (-52.3091, 54.6138) -> (-59.1525, 53.5331)
  line L612 (-59.1525, 53.5331) -> (-63.5101, 58.9193)
  line L613 (-63.5101, 58.9193) -> (-61.0243, 65.3862)
  line L614 (-61.0243, 65.3862) -> (-54.1809, 66.4669)
  line L615 (-54.1809, 66.4669) -> (-49.8233, 61.0807)
  line L616 (-49.8233, 93.0807) -> (-52.3091, 86.6138)
  line L617 (-52.3091, 86.6138) -> (-59.1525, 85.5331)
  line L618 (-59.1525, 85.5331) -> (-63.5101, 90.9193)
  line L619 (-63.5101, 90.9193) -> (-61.0243, 97.3862)
  line L620 (-61.0243, 97.3862) -> (-54.1809, 98.4669)
  line L621 (-54.1809, 98.4669) -> (-49.8233, 93.0807)
  line L622 (-49.8233, 125.0807) -> (-52.3091, 118.6138)
  line L623 (-52.3091, 118.6138) -> (-59.1525, 117.5331)
  line L624 (-59.1525, 117.5331) -> (-63.5101, 122.9193)
  line L625 (-63.5101, 122.9193) -> (-61.0243, 129.3862)
  line L626 (-61.0243, 129.3862) -> (-54.1809, 130.4669)
  line L627 (-54.1809, 130.4669) -> (-49.8233, 125.0807)
  line L628 (-63.1566, -18.9193) -> (-65.6424, -25.3862)
  line L629 (-65.6424, -25.3862) -> (-72.4858, -26.4669)
  line L630 (-72.4858, -26.4669) -> (-76.8434, -21.0807)
  line L631 (-76.8434, -21.0807) -> (-74.3576, -14.6138)
  line L632 (-74.3576, -14.6138) -> (-67.5142, -13.5331)
  line L633 (-67.5142, -13.5331) -> (-63.1566, -18.9193)
  line L634 (-63.1566, 13.0807) -> (-65.6424, 6.6138)
  line L635 (-65.6424, 6.6138) -> (-72.4858, 5.5331)
  line L636 (-72.4858, 5.5331) -> (-76.8434, 10.9193)
  line L637 (-76.8434, 10.9193) -> (-74.3576, 17.3862)
  line L638 (-74.3576, 17.3862) -> (-67.5142, 18.4669)
  line L639 (-67.5142, 18.4669) -> (-63.1566, 13.0807)
  line L640 (-63.1566, 45.0807) -> (-65.6424, 38.6138)
  line L641 (-65.6424, 38.6138) -> (-72.4858, 37.5331)
  line L642 (-72.4858, 37.5331) -> (-76.8434, 42.9193)
  line L643 (-76.8434, 42.9193) -> (-74.3576, 49.3862)
  line L644 (-74.3576, 49.3862) -> (-67.5142, 50.4669)
  line L645 (-67.5142, 50.4669) -> (-63.1566, 45.0807)
  line L646 (-63.1566, 77.0807) -> (-65.6424, 70.6138)
  line L647 (-65.6424, 70.6138) -> (-72.4858, 69.5331)
  line L648 (-72.4858, 69.5331) -> (-76.8434, 74.9193)
  line L649 (-76.8434, 74.9193) -> (-74.3576, 81.3862)
  line L650 (-74.3576, 81.3862) -> (-67.5142, 82.4669)
  line L651 (-67.5142, 82.4669) -> (-63.1566, 77.0807)
  line L652 (-63.1566, 109.0807) -> (-65.6424, 102.6138)
  line L653 (-65.6424, 102.6138) -> (-72.4858, 101.5331)
  line L654 (-72.4858, 101.5331) -> (-76.8434, 106.9193)
  line L655 (-76.8434, 106.9193) -> (-74.3576, 113.3862)
  line L656 (-74.3576, 113.3862) -> (-67.5142, 114.4669)
  line L657 (-67.5142, 114.4669) -> (-63.1566, 109.0807)
  line L658 (-63.1566, 141.0807) -> (-65.6424, 134.6138)
  line L659 (-65.6424, 134.6138) -> (-72.4858, 133.5331)
  line L660 (-72.4858, 133.5331) -> (-76.8434, 138.9193)
  line L661 (-76.8434, 138.9193) -> (-74.3576, 145.3862)
  line L662 (-74.3576, 145.3862) -> (-67.5142, 146.4669)
  line L663 (-67.5142, 146.4669) -> (-63.1566, 141.0807)
  line L664 (-11, 37.5) -> (-8.5, 37.5)
  line L665 (-8.5, 37.5) -> (-8.5, 35)
  line L666 (-8.5, 35) -> (-11, 35)
  line L667 (-11, 35) -> (-11, 37.5)
  line L668 (2.5, 37.5) -> (5, 37.5)
  line L669 (5, 37.5) -> (5, 35)
  line L670 (5, 35) -> (2.5, 35)
  line L671 (2.5, 35) -> (2.5, 37.5)
  dimension "d23" = 2.5
  dimension "d24" = 2.5
  dimension "d25" = 2.5
  dimension "d26" = 2.5
  constraint horizontal L664
  constraint vertical L665
  constraint horizontal L666
  constraint vertical L667
  constraint horizontal L668
  constraint vertical L669
  constraint horizontal L670
  constraint vertical L671
  measures "d23" distance of L664.start L664.end
  measures "d24" distance of L664.start L666.end
  measures "d25" distance of L668.start L668.end
  measures "d26" distance of L668.start L670.end
extrude "Extrude5" add sketch "Sketch4" along normal blind 70 contours L664 L665 L666 L667 | L668 L669 L670 L671 bodies 1